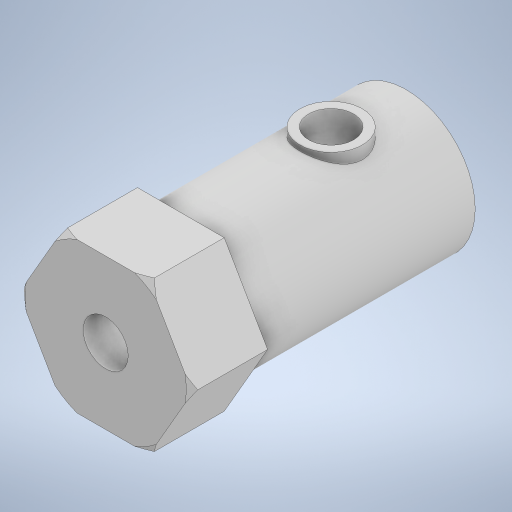
# Autodesk Inventor part: PIN
Saved by Autodesk Inventor 2024 (Build 280153000, 153)
## iProperties
Created: 2023-10-30
Part Number: PIN
Material: Generic
Document SubType Name: Modeling
Designer: jebes windows
Density: 1 g/cm^3
Appearance: Default
Author: jebes windows
## iProperties of the stored document PIN_3DPrint.ipt
Created: 2023-10-30
Part Number: PIN_3DPrint
Material: Generic
Document SubType Name: Modeling
Designer: jebes windows
Density: 1 g/cm^3
Appearance: Default
Author: jebes windows
Autodesk Inventor part; units mm, degrees
ref_plane "YZ Plane" through (0, 0, 0) normal (1, 0, 0) x (0, 1, 0)
ref_plane "XZ Plane" through (0, 0, 0) normal (0, 1, 0) x (-1, 0, 0)
ref_plane "XY Plane" through (0, 0, 0) normal (0, 0, 1) x (1, 0, 0)
sketch "Sketch7" plane through (0, 0, 0) normal (0, 1, 0) x (-1, 0, 0)
  line L0 (-3.4641, -6) -> (-6.9282, 0)
  line L1 (-6.9282, 0) -> (-3.4641, 6)
  line L2 (-3.4641, 6) -> (3.4641, 6)
  line L3 (3.4641, 6) -> (6.9282, 0)
  line L4 (6.9282, 0) -> (3.4641, -6)
  line L5 (3.4641, -6) -> (-3.4641, -6)
  point P0 (0, 0)
  point P1 (0, 0)
  point P2 (0, -6)
  dimension "d24" = 12
  constraints: 12 end point, 1 coincident, 1 horizontal alignment, 1 midpoint, 13 other
  measures "d24" distance from line of point (0, -6) L2
extrude "Extrusion6" add sketch "Sketch7" along normal blind 6
sketch "Sketch8" plane through (0, 6, 0) normal (0, 1, 0) x (1, 0, 0)
  circle A0 centre (0, 0) radius 5.5
  circle A1 centre (0, 0) radius 2.575
  line L0 (-0.1332, 2.5716) -> (-0.1332, -1.9284)
  line L1 (-0.1332, -1.9284) -> (-1.7064, -1.9284)
  line L2 (-0.1332, -1.9284) -> (1.7064, -1.9284)
  dimension "d27" = 11
  dimension "d28" = 5.15
  dimension "d29" = 4.5
  dimension "d30" = 1.5732
  constraints: 6 end point, 3 point on circle, 2 centre point, 2 coincident, 1 perpendicular, 1 point on line, 1 vertical
  measures "d27" diameter of A0
  measures "d28" diameter of A1
  measures "d29" distance of L0.start L0.end
  measures "d30" distance of L0.end L1.end
extrude "Extrusion7" add sketch "Sketch8" along normal blind 18 contours A0 | A1 L1 L2
sketch "Sketch9" plane through (0, 0, 0) normal (0, 0, 1) x (1, 0, 0)
  line L0 (6.9282, 0) -> (3.4641, 0) projected
  line L1 (6.9282, 0) -> (6.4282, 0)
  line L2 (6.8032, 0.3147) -> (6.4282, 0)
  line L3 (6.9282, 0) -> (6.9282, 0.3868)
  line L4 (0, -4.8) -> (0, 28.8) projected
  line L5 (6.8032, 0.3147) -> (6.9282, 0.4195)
  line L6 (6.9282, 0.4195) -> (6.9282, 0.3868)
  point P0 (0, 0)
  dimension "d33" = 0.5
  dimension "d35" = 40
  dimension "d39" = 0.125
  dimension "d40" = 0.1049
  constraints: 10 end point, 2 vertical, 1 point on line
  measures "d33" distance of L0.start L1.end
  measures "d35" angle of L2 L0
  measures "d39" horizontal distance of L2.start L5.end
  measures "d40" vertical distance of L2.start L5.end
revolve "Revolution1" cut sketch "Sketch9" angle 360 about axis through (0, -10, 0) along (0, 1, 0)
chamfer "Chamfer3" distance 1 angle 45 2 edges at (0, 24, -2.575) (0, 24, 1.9284)
sketch "Sketch10" plane through (0, 0, 0) normal (0, -1, 0) x (1, 0, 0)
  circle A0 centre (0, 0) radius 1.8
  dimension "d44" = 3.6
  constraints: 1 centre point, 1 coincident
  measures "d44" diameter of A0
extrude "Extrusion8" cut sketch "Sketch10" against normal through all
sketch "Sketch13" plane through (1.7064, 6, 1.9284) normal (0, 0, -1) x (-1, 0, 0)
  circle A0 centre (1.7064, 12) radius 1.8
  point P0 (1.7064, -6)
  dimension "d55" = 3.6
  dimension "d56" = 18
  dimension "d57" = 0
  constraints: 1 centre point
  measures "d55" diameter of A0
  measures "d56" distance of A0.centre point (1.706, -6)
  measures "d57" horizontal distance of point (1.706, -6) A0.centre
extrude "Extrusion11" cut sketch "Sketch13" against normal through all
ref_plane "Work Plane2" through (1.7064, 6, 5.9284) normal (0, 0, -1) x (-1, 0, 0)
sketch "Sketch14" plane through (1.7064, 6, 5.9284) normal (0, 0, -1) x (-1, 0, 0)
  spline S0 degree 8 poles (3.5064, 12) (3.5064, 12.1901) (3.4834, 12.3798) (3.4377, 12.5672) (3.3691, 12.7503) (3.2769, 12.9271) (3.1607, 13.0947) (3.0198, 13.2496) (2.7182, 13.499) (2.5613, 13.6034) (2.3851, 13.6923) (2.1931, 13.7603) (1.99, 13.8033) (1.7813, 13.819) (1.5725, 13.8069) (1.1492, 13.7262) (0.9448, 13.6548) (0.7585, 13.5594) (0.5918, 13.4445) (0.4454, 13.3144) (0.3197, 13.1725) (0.2144, 13.0225) (0.0308, 12.6885) (-0.0422, 12.5008) (-0.0906, 12.3073) (-0.1146, 12.1105) (-0.1143, 11.9127) (-0.0899, 11.7163) (-0.041, 11.5236) (0.0949, 11.1805) (0.1748, 11.0279) (0.2727, 10.8814) (0.3891, 10.7428) (0.5244, 10.6146) (0.6789, 10.4998) (0.8523, 10.4022) (1.2226, 10.2556) (1.417, 10.2039) (1.6217, 10.1768) (1.8302, 10.1772) (2.0358, 10.2054) (2.2319, 10.2593) (2.4126, 10.3342) (2.8114, 10.5534) (3.0139, 10.7181) (3.1802, 10.9062) (3.3115, 11.1105) (3.409, 11.3257) (3.4738, 11.5476) (3.5064, 11.7733) (3.5064, 12) knots 0 0 0 0 0 0 0 0 0 0.152782 0.152782 0.152782 0.152782 0.152782 0.152782 0.152782 0.27746 0.27746 0.27746 0.27746 0.27746 0.27746 0.27746 0.412202 0.412202 0.412202 0.412202 0.412202 0.412202 0.412202 0.567191 0.567191 0.567191 0.567191 0.567191 0.567191 0.567191 0.697775 0.697775 0.697775 0.697775 0.697775 0.697775 0.697775 0.819734 0.819734 0.819734 0.819734 0.819734 0.819734 0.819734 1 1 1 1 1 1 1 1 1 projected
  circle A0 centre (1.7064, 12) radius 2.5
  line L0 (4.0133, -6) -> (-0.6005, -6) projected
  point P0 (1.7064, -6)
  point P1 (1.7064, -6)
  point P2 (1.7064, -6)
  dimension "d61" = 5
  dimension "d62" = 18
  constraints: 2 midpoint, 1 centre point, 1 vertical alignment, 1 other
  measures "d61" diameter of A0
  measures "d62" distance of point (1.706, -6) A0.centre
extrude "Extrusion12" add sketch "Sketch14" along normal up to surface round surface about axis through (0, 6, 0) along (0, 1, 0) radius 5.5 far side no
body "Solid2"
